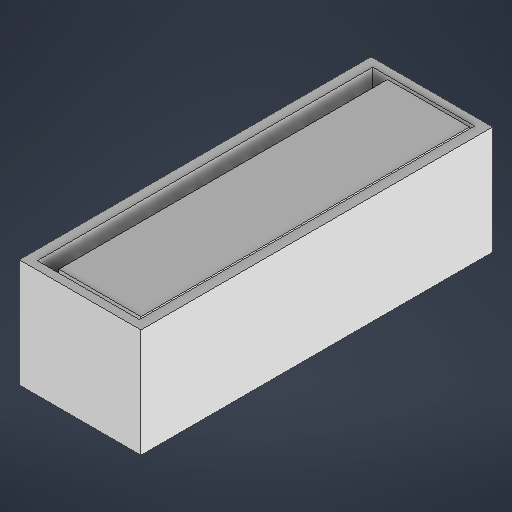
# Autodesk Inventor part: camerahouse
Saved by Autodesk Inventor 2026.2 (Build 302298000, 298)
## iProperties
Created: 2026-02-10
Part Number: camerahouse
Material: Generic
Document SubType Name: Modeling
Designer: small.ab
Density: 1 g/cm^3
Appearance: Default
Author: small.ab
Autodesk Inventor part; units mm, degrees
ref_plane "YZ Plane" through (0, 0, 0) normal (1, 0, 0) x (0, 1, 0)
ref_plane "XZ Plane" through (0, 0, 0) normal (0, 1, 0) x (-1, 0, 0)
ref_plane "XY Plane" through (0, 0, 0) normal (0, 0, 1) x (1, 0, 0)
sketch "Sketch1" plane through (0, 0, 0) normal (0, 0, 1) x (1, 0, 0)
  line L0 (0, 0) -> (100, 0)
  line L1 (100, 0) -> (100, 25)
  line L2 (100, 25) -> (0, 25)
  line L3 (0, 25) -> (0, 0)
  dimension "cameralength" = 100
  dimension "cameraheight" = 25
  constraints: 8 end point, 2 parallel, 1 horizontal, 1 perpendicular
  measures "cameralength" distance of L2.end L1.end
  measures "cameraheight" distance of L0.end L1.end
extrude "Extrusion1" add sketch "Sketch1" along normal blind 30
sketch "Sketch2" plane through (0, 0, 0) normal (0, -1, 0) x (1, 0, 0)
  line L0 (0, 0) -> (0, 30) projected
  line L1 (100, 30) -> (0, 30) projected
  line L2 (100, 0) -> (100, 30) projected
  circle A0 centre (49.9989, 14.9997) radius 9.6139
  dimension "bottomdiameter" = 19.2278
  constraints: 1 centre point
  measures "bottomdiameter" diameter of A0
extrude "Extrusion2" add sketch "Sketch2" along normal blind 5
sketch "Sketch3" plane through (49.9989, 25, 30) normal (0, 0, 1) x (1, 0, 0)
  line L0 (53.5011, -33.5) -> (-53.4989, -33.5)
  line L1 (-53.4989, -33.5) -> (-53.4989, 3.5)
  line L2 (-53.4989, 3.5) -> (53.5011, 3.5)
  line L3 (53.5011, 3.5) -> (53.5011, -33.5)
  line L4 (53.5011, -33.5) -> (-53.4989, 3.5) construction
  line L5 (-53.4989, -33.5) -> (53.5011, 3.5) construction
  line L6 (50.0011, -25) -> (50.0011, -25) projected
  line L7 (-49.9989, -25) -> (50.0011, -25) projected
  line L8 (-49.9989, -25) -> (50.0011, -25) projected
  line L9 (50.0011, -25) -> (50.0011, -25) projected
  line L10 (-49.9989, -25) -> (50.0011, -25) projected
  line L11 (-49.9989, -25) -> (-49.9989, -25) projected
  line L12 (-50.9989, 0.5) -> (51.0011, 0.5)
  line L13 (51.0011, 0.5) -> (51.0011, -30.5)
  line L14 (51.0011, -30.5) -> (-50.9989, -30.5)
  line L15 (-50.9989, -30.5) -> (-50.9989, 0.5)
  line L16 (-50.9989, 0.5) -> (51.0011, -30.5) construction
  line L17 (51.0011, 0.5) -> (-50.9989, -30.5) construction
  line L18 (50.0011, -25) -> (50.0011, 0) projected
  line L19 (-9.6139, -30) -> (9.6139, -30) projected
  line L20 (9.6139, -25) -> (-9.6139, -25) projected
  line L21 (50.0011, 0) -> (-49.9989, 0) projected
  point P0 (0.0011, -15)
  point P1 (50.0011, 15.0003)
  point P2 (-49.9989, -14.9997)
  dimension "bottomheight" = 5
  dimension "d7" = 37
  dimension "d8" = 107
  dimension "d9" = 3.5
  dimension "d16" = 1
  dimension "d18" = 0.5
  dimension "d19" = 31
  dimension "d20" = 3
  constraints: 24 end point, 4 midpoint, 4 parallel, 2 horizontal, 2 perpendicular
  measures "d7" distance between parallel lines of L0 L2
  measures "d8" distance between parallel lines of L3 L1
  measures "d9" distance between parallel lines of L3 L6
  measures "d16" distance between parallel lines of L13 L18
  measures "d18" distance between parallel lines of L12 L21
  measures "d19" distance between parallel lines of L12 L14
  measures "d20" distance between parallel lines of L14 L0
extrude "Extrusion3" add sketch "Sketch3" against normal up to surface (30 mm away) separate body
sketch "Sketch4" plane through (49.9989, 25, 30) normal (0, 0, 1) x (1, 0, 0)
  line L0 (53.5011, 3.5) -> (-53.4989, 3.5) projected
  line L1 (-53.4989, 3.5) -> (-53.4989, -33.5) projected
  line L2 (-53.4989, -33.5) -> (53.5011, -33.5) projected
  line L3 (53.5011, -33.5) -> (53.5011, 3.5) projected
  line L4 (-50.9989, 0.5) -> (51.0011, 0.5) projected
  line L5 (51.0011, 0.5) -> (51.0011, -30.5) projected
  line L6 (51.0011, -30.5) -> (-50.9989, -30.5) projected
  line L7 (-50.9989, -30.5) -> (-50.9989, 0.5) projected
  line L8 (-53.4989, 3.5) -> (53.5011, 3.5)
  line L9 (53.5011, 3.5) -> (53.5011, -33.5)
  line L10 (53.5011, -33.5) -> (-53.4989, -33.5)
  line L11 (-53.4989, -33.5) -> (-53.4989, 3.5)
  circle A0 centre (0.0011, -12.5) radius 10
  line L12 (50.0011, -25) -> (50.0011, 0) projected
  line L13 (50.0011, 0) -> (-49.9989, 0) projected
  line L14 (-49.9989, 0) -> (-49.9989, -25) projected
  line L15 (-49.9989, -25) -> (50.0011, -25) projected
  dimension "cordhole" = 20
  constraints: 8 end point, 2 parallel, 1 centre point, 1 horizontal, 1 perpendicular
  measures "cordhole" diameter of A0
extrude "Extrusion4" add sketch "Sketch4" along normal blind 3 contours L3 L2 L1 L0 | L4 L5 L6 L7 | L15 L14 L13 L12 bodies 2
equation "\"d7\" = 2 * wallthickness + cameraheight + bottomheight + tolerance"
equation "\"d8\" = 2 * wallthickness + cameralength + tolerance"
equation "\"d9\" = wallthickness + 0.5 * tolerance"
equation "\"d16\" = tolerance"
equation "\"d18\" = 0.5 * tolerance"
equation "\"d19\" = bottomheight + cameraheight + tolerance"
equation "\"d22\" = wallthickness"
equation "\"tolerance\" = 1"
equation "\"wallthickness\" = 3"
body "Solid2"
